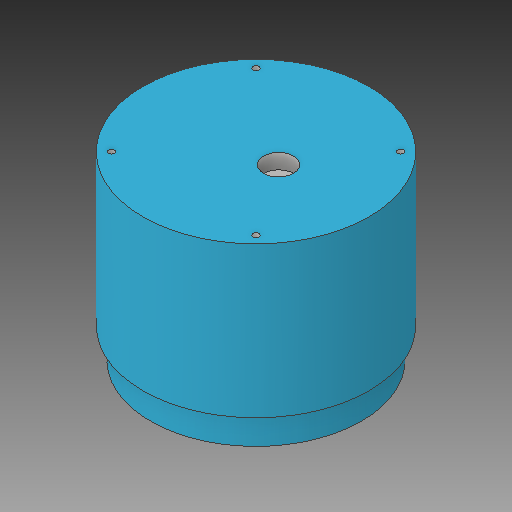
# Autodesk Inventor part: 바텀(상)
Saved by Autodesk Inventor 2019 (Build 230136000, 136)
## iProperties
Created: 2018-04-02
Part Number: 바텀(상)
Material: 일반
Document SubType Name: Modeling
Designer: CK
Density: 1 g/cm^3
Appearance: 기본값
Mass: 608.857 g
Surface Area: 1370.4 cm^2
Volume: 608.857 cm^3
Author: CK
Autodesk Inventor part; units mm, degrees
ref_plane "YZ Plane" through (0, 0, 0) normal (1, 0, 0) x (0, 1, 0)
ref_plane "XY Plane" through (0, 0, 0) normal (0, 0, 1) x (1, 0, 0)
sketch "스케치2" plane through (0, 0, 0) normal (0, 1, 0) x (-1, 0, 0)
  circle A0 centre (0, 0) radius 75
  dimension "d1" = 150
  constraints: 1 centre point, 1 coincident
  measures "d1" diameter of A0
extrude "돌출1" add sketch "스케치2" along normal blind 100
shell "쉘1" thickness 10 removed faces 1 at (-17.7208, 0, 28.0232)
sketch "스케치4" plane through (0, 0, 0) normal (0, -1, 0) x (1, 0, 0)
  circle A0 centre (0, 0) radius 65
  circle A1 centre (0, 0) radius 70
  dimension "d10" = 140
  constraints: 2 centre point, 2 coincident
  measures "d10" diameter of A1
extrude "돌출3" add sketch "스케치4" along normal blind 20
ref_plane "작업 평면1" through (0, -20, 0) normal (0, 1, 0) x (-1, 0, 0)
sketch "스케치5" plane through (0, -20, 0) normal (0, 1, 0) x (-1, 0, 0)
  circle A0 centre (-67.5, 0) radius 1.35
  circle A1 centre (0, -67.5) radius 1.35
  circle A2 centre (67.5, 0) radius 1.35
  circle A3 centre (0, 67.5) radius 1.35
  point P0 (0, 0)
  point P1 (0, -67.5)
  point P2 (0, 0)
  point P3 (67.5, 0)
  point P4 (0, 0)
  point P5 (0, 67.5)
  point P6 (0, 0)
  point P7 (0, 0)
  dimension "d17" = 360
  dimension "d71" = 360
  constraints: 4 centre point, 1 coincident, 18 other
sketch "스케치7" plane through (0, 100, 0) normal (0, 1, 0) x (1, 0, 0)
  circle A0 centre (15, 0) radius 10
  point P0 (0, 0)
  dimension "d45" = 20
  dimension "d46" = 15
  constraints: 1 centre point
  measures "d45" diameter of A0
  measures "d46" distance of point (0, 0) A0.centre
extrude "돌출4" cut sketch "스케치7" against normal blind 10
sketch "스케치8" plane through (0, 0, 0) normal (1, 0, 0) x (0, 1, 0)
  circle A0 centre (50, 0) radius 8.5
  line L0 (0, 75) -> (0, -75) projected
  point P0 (0, 0)
  dimension "d30" = 17
  dimension "d31" = 50
  constraints: 1 centre point
  measures "d30" diameter of A0
  measures "d31" distance from line of L0 A0.centre
extrude "돌출5" cut sketch "스케치8" against normal through all
sketch "스케치12" plane through (0, 100, 0) normal (0, 1, 0) x (1, 0, 0)
  circle A0 centre (15, 0) radius 10 projected
  circle A1 centre (48, -48) radius 2
  circle A2 centre (-48, -48) radius 2
  circle A3 centre (48, 48) radius 2
  circle A4 centre (-48, 48) radius 2
  line L0 (48, 48) -> (-48, -48) construction
  line L1 (-48, 48) -> (48, -48) construction
  point P0 (0, 0)
  dimension "d66" = 4
  dimension "d75" = 96
  dimension "d76" = 96
  constraints: 4 centre point, 4 coincident, 4 end point, 2 midpoint
  measures "d66" diameter of A1
  measures "d75" distance of L1.end L0.end
  measures "d76" distance of L0.end L1.start
extrude "돌출8" cut sketch "스케치12" against normal blind 10 contours A1 | A2 | A3 | A4
extrude "돌출9" cut sketch "스케치5" along normal blind 8
